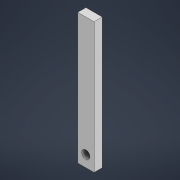
# Autodesk Inventor part: Circle_TestFit_V1
Saved by Autodesk Inventor 2022 (Build 260153000, 153)
## iProperties
Created: 2023-05-10
Part Number: Circle_TestFit_V1
Material: Generic
Document SubType Name: Modeling
Designer: Karl Spiteri
Density: 1 g/cm^3
Appearance: Default
Author: Karl Spiteri
Autodesk Inventor part; units mm, degrees
ref_plane "YZ Plane" through (0, 0, 0) normal (1, 0, 0) x (0, 1, 0)
ref_plane "XZ Plane" through (0, 0, 0) normal (0, 1, 0) x (-1, 0, 0)
ref_plane "XY Plane" through (0, 0, 0) normal (0, 0, 1) x (1, 0, 0)
sketch "Sketch2" plane through (0, 0, 0) normal (0, 0, 1) x (1, 0, 0)
  line L0 (0, 0) -> (-10, 0)
  line L1 (-10, 0) -> (-10, 80)
  line L2 (-10, 80) -> (0, 80)
  line L3 (0, 80) -> (0, 0)
  point P0 (-5, 18)
  dimension "d4" = 10
  dimension "d5" = 80
  constraints: 8 end point, 2 parallel, 1 horizontal, 1 perpendicular
  measures "d4" distance of L1.end L2.end
  measures "d5" distance of L0.end L1.end
extrude "Extrusion2" add sketch "Sketch2" along normal blind 5
sketch "Sketch3" plane through (0, 0, 5) normal (0, 0, 1) x (1, 0, 0)
  point P0 (0, 0)
  point P1 (-5, 7)
hole "Hole2" at (-5, 7, 5) direction (0, 0, -1) diameter 5 depth 5
body "Solid2"
